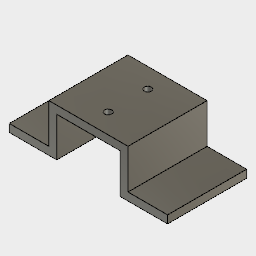
psu-stand (Autodesk Fusion 360 design; units mm, degrees)
Autodesk Fusion 360 part; units mm, degrees
sketch "Sketch9" plane through (0, 0, 0) normal (0, 0, 1) x (1, 0, 0)
  line L0 (0, 50) -> (50, 50)
  line L1 (50, 50) -> (50, 0)
  line L2 (50, 0) -> (0, 0)
  line L3 (0, 0) -> (0, 50)
  line L4 (-25, 50) -> (0, 50)
  line L5 (0, 50) -> (0, 0)
  line L6 (0, 0) -> (-25, 0)
  line L7 (-25, 0) -> (-25, 50)
  line L8 (50, 50) -> (75, 50)
  line L9 (75, 50) -> (75, 0)
  line L10 (75, 0) -> (50, 0)
  line L11 (50, 0) -> (50, 50)
  dimension "d34" = 50
  dimension "d35" = 50
  dimension "d36" = 25
  dimension "d37" = 50
  measures "d34" distance of L0.start L0.end
  measures "d35" distance of L0.start L2.end
  measures "d36" distance of L0.end L8.end
  measures "d37" distance of L8.end L9.end
extrude "Extrude5" add sketch "Sketch9" along normal blind 30 contours L0 L1 L2 L3 L5 L11
extrude "Extrude6" add sketch "Sketch9" along normal blind 5 contours L1 L8 L9 L10 L11
extrude "Extrude7" add sketch "Sketch9" along normal blind 5 contours L3 L4 L5 L6 L7
sketch "Sketch12" plane through (0, 0, 0) normal (0, 1, 0) x (1, 0, 0)
  line L0 (5, -25) -> (45, -25)
  line L1 (45, -25) -> (45, 0)
  line L2 (45, 0) -> (5, 0)
  line L3 (5, 0) -> (5, -25)
  line L4 (50, 0) -> (0, 0)
  line L5 (75, 0) -> (-25, 0)
  line L6 (-25, 0) -> (75, 0)
  line L7 (0, -30) -> (50, -30)
  line L8 (0, -5) -> (0, -30)
  line L9 (50, -5) -> (50, -30)
  dimension "d44" = 5
  dimension "d45" = 5
  dimension "d46" = 5
  measures "d44" distance of L0 L7
  measures "d45" distance of L3 L8
  measures "d46" distance of L1 L9
extrude "Extrude8" cut sketch "Sketch12" along normal through all
sketch "Sketch13" plane through (0, 0, 30) normal (0, 0, 1) x (-1, 0, 0)
  line L0 (0, -50) -> (0, 0)
  line L1 (0, 0) -> (-50, 0)
  line L2 (-50, 0) -> (-50, -50)
  line L3 (-50, -50) -> (0, -50)
  circle A0 centre (-25, -12.5) radius 2.25
  circle A1 centre (-25, -37.5) radius 2.25
  dimension "d48" = 4.5
  dimension "d49" = 4.5
  dimension "d50" = 25
  dimension "d51" = 25
  dimension "d52" = 12.5
  measures "d48" diameter of A0
  measures "d49" diameter of A1
  measures "d50" distance of A0.centre A1.centre
  measures "d51" distance of L0 A0.centre
  measures "d52" distance of L1 A0.centre
extrude "Extrude9" cut sketch "Sketch13" against normal through all contours A0
extrude "Extrude10" cut sketch "Sketch13" against normal through all contours A1
